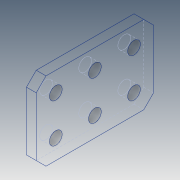
# Autodesk Inventor part: 200-40-BOGIE-CONNECTOR-06
Saved by Autodesk Inventor 2018.2 (Build 222227000, 227)
## iProperties
Manager: feesmrt
Company: FRANCOR
Part Number: 200-40-BOGIE-CONNECTOR-06
Project: Rescue Robot
Cost Center: -
Material: Aluminium 6061
Document SubType Name: Modeling
Designer: feesmrt
Engineer: feesmrt
Authority: feesmrt
Density: 2.7 g/cm^3
Appearance: Aluminium - flach
Description: Bogie Connector Verstärkungsplatte
Stock Number: 200-40-BOGIE-CONNECTOR-06
Subject: Rescue Robot
Author: feesmrt
Revision Number: 1
Title: Bogie Connector Verstärkungsplatte
Autodesk Inventor part; units mm, degrees
ref_plane "YZ Plane" through (0, 0, 0) normal (1, 0, 0) x (0, 1, 0)
ref_plane "XZ Plane" through (0, 0, 0) normal (0, 1, 0) x (-1, 0, 0)
ref_plane "XY Plane" through (0, 0, 0) normal (0, 0, 1) x (1, 0, 0)
sketch "Skizze1" plane through (0, 0, 0) normal (1, 0, 0) x (0, 1, 0)
  line L0 (0, 28) -> (0, -28) construction
  line L1 (-42, 0) -> (42, 0) construction
  line L2 (-30, -20) -> (30, -20)
  line L3 (30, -20) -> (30, 20)
  line L4 (30, 20) -> (-30, 20)
  line L5 (-30, 20) -> (-30, -20)
  line L6 (-30, -20) -> (30, 20) construction
  line L7 (30, -20) -> (-30, 20) construction
  point P0 (0, 0)
  dimension "d0" = 60
  dimension "d1" = 40
  constraints: 12 end point, 2 midpoint, 2 parallel, 1 horizontal, 1 perpendicular
  measures "d0" distance between parallel lines of L3 L5
  measures "d1" distance of L2.end L3.end
extrude "Grundkörper" add sketch "Skizze1" along normal mid plane 5
sketch "Skizze2" plane through (2.5, 0, 0) normal (1, 0, 0) x (0, 0, -1)
  line L0 (-20, 30) -> (-20, -30) construction
  line L1 (20, -30) -> (20, 30) construction
  line L2 (20, 30) -> (-20, 30) construction
  line L3 (-20, 30) -> (-20, -30) construction
  line L4 (-20, -30) -> (20, -30) construction
  line L5 (-20, -20) -> (20, -20) construction
  line L6 (0, -42) -> (0, 42) construction
  line L7 (20, 30) -> (-20, 30) projected
  line L8 (-10, 30) -> (-10, 0) construction
  line L9 (-28, 0) -> (28, 0) construction
  line L10 (10, 30) -> (10, 0) construction
  point P0 (0, 0)
  point P1 (-10, -20)
  point P2 (10, -20)
  point P3 (-10, 0)
  point P4 (-10, 20)
  point P5 (10, 0)
  point P6 (10, 20)
  dimension "d4" = 10
  dimension "d5" = 20
  dimension "d18" = 20
  dimension "d19" = 10
  dimension "d20" = 20
  constraints: 9 point on line, 6 end point, 5 symmetric about line, 2 perpendicular
  measures "d4" distance between parallel lines of L4 L5
  measures "d5" distance of point (10, -20) point (-10, -20)
  measures "d18" distance between parallel lines of L10 L8
  measures "d19" distance from line of L2 point (-10, 20)
  measures "d20" distance of point (-10, 0) point (-10, 20)
hole "BOH_M6" at (2.5, -20, 10) at (2.5, -20, -10) at (2.5, 0, 10) at (2.5, 20, 10) at (2.5, 20, -10) at (2.5, 0, -10) direction (-1, 0, 0) diameter 6.5 end through all
chamfer "Fase_Allgemein" distance 5 angle 45 4 edges at (0, -30, 20) (0, -30, -20) (0, 30, 20) (0, 30, -20)
equation "\"d5\" = d20"
